Autodesk Inventor part; units mm, degrees
(part 2 of 2)
sketch "スケッチ14" plane through (196, 25, -10) normal (1, 0, 0) x (0, 0, -1)
  line L0 (16, -8.5343) -> (12, -8.5343) projected
  line L1 (16, 0) -> (16, -8.5343) projected
  line L2 (0, 0) -> (16, 0) projected
  line L3 (0, 0) -> (0, -4) projected
  line L4 (12, -4) -> (0, -4) projected
  line L5 (12, -8.5343) -> (12, -4) projected
  line L6 (12, -41.4657) -> (16, -41.4657) projected
  line L7 (12, -46) -> (12, -41.4657) projected
  line L8 (0, -46) -> (12, -46) projected
  line L9 (0, -46) -> (0, -50) projected
  line L10 (16, -50) -> (0, -50) projected
  line L11 (16, -41.4657) -> (16, -50) projected
  line L12 (16, -41.4657) -> (16, -50) projected
  line L13 (12, -8.5343) -> (16, -8.5343)
  line L14 (16, -8.5343) -> (16, -41.4657)
  line L15 (16, -41.4657) -> (12, -41.4657)
  line L16 (12, -41.4657) -> (12, -8.5343)
  point P0 (-10, -25)
  constraints: 8 end point, 2 parallel, 1 horizontal, 1 perpendicular
extrude "押し出し22" add sketch "スケッチ14" against normal blind 4 contours L14 L6 L16 L0
mirror "ミラー4" about plane through (0, 0, 0) normal (1, 0, 0) of "押し出し19", "押し出し16", "押し出し20", "押し出し18", "押し出し17"
sketch "スケッチ15" plane through (-196, 16.4657, -26) normal (-1, 0, 0) x (0, 0, 1)
  line L0 (4, 0) -> (0, 0) projected
  line L1 (4, 4.5343) -> (4, 0) projected
  line L2 (16, 4.5343) -> (4, 4.5343) projected
  line L3 (16, 8.5343) -> (16, 4.5343) projected
  line L4 (0, 8.5343) -> (16, 8.5343) projected
  line L5 (0, 0) -> (0, 8.5343) projected
  line L6 (0, -32.9313) -> (4, -32.9313) projected
  line L7 (0, -41.4657) -> (0, -32.9313) projected
  line L8 (16, -41.4657) -> (0, -41.4657) projected
  line L9 (16, -37.4657) -> (16, -41.4657) projected
  line L10 (4, -37.4657) -> (16, -37.4657) projected
  line L11 (4, -32.9313) -> (4, -37.4657) projected
  line L12 (4, 0) -> (0, 0)
  line L13 (0, 0) -> (0, -32.9313)
  line L14 (0, -32.9313) -> (4, -32.9313)
  line L15 (4, -32.9313) -> (4, 0)
  point P0 (26, -16.4657)
  constraints: 8 end point, 2 parallel, 1 horizontal, 1 perpendicular
extrude "押し出し23" add sketch "スケッチ15" against normal blind 4 contours L15 L6 L13 L0
